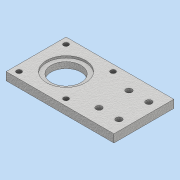
# Autodesk Inventor part: Uchwyt silnika krokowego osi Y - płaski
Saved by Autodesk Inventor 2018 (Build 220112000, 112)
## iProperties
Created: 2019-01-31
Part Number: Uchwyt silnika krokowego osi Y - płaski
Material: Ogólny
Document SubType Name: Modeling
Designer: Dawid
Density: 1 g/cm^3
Appearance: Aluminium odlewane
Author: Dawid
Autodesk Inventor part; units mm, degrees
ref_plane "YZ Plane" through (0, 0, 0) normal (1, 0, 0) x (0, 1, 0)
ref_plane "XZ Plane" through (0, 0, 0) normal (0, 1, 0) x (-1, 0, 0)
ref_plane "XY Plane" through (0, 0, 0) normal (0, 0, 1) x (1, 0, 0)
sketch "Szkic1" plane through (0, 0, 0) normal (0, 0, 1) x (1, 0, 0)
  circle A0 centre (30, 30) radius 15
  circle A1 centre (53.57, 6.43) radius 2.5
  circle A2 centre (6.43, 53.57) radius 2.5
  circle A3 centre (6.43, 6.43) radius 2.5
  circle A4 centre (53.57, 53.57) radius 2.5
  line L0 (0, 60) -> (0, 0)
  line L1 (0, 0) -> (78, 0)
  circle A5 centre (78, 45) radius 3
  circle A6 centre (98, 45) radius 3
  circle A7 centre (98, 15) radius 3
  circle A8 centre (78, 15) radius 3
  line L2 (108, 60) -> (108, 0)
  line L3 (0, 60) -> (108, 60)
  line L4 (108, 0) -> (78, 0)
  point P0 (35, 30)
  dimension "d12" = 6.43
  dimension "d13" = 6.43
  dimension "d14" = 47.14
  dimension "d15" = 47.14
  dimension "d16" = 30
  dimension "d17" = 10
  dimension "d18" = 10
  dimension "d19" = 30
  dimension "d20" = 30
  dimension "d21" = 108
  constraints: 10 end point, 9 centre point, 1 horizontal, 1 parallel
  measures "d12" distance from line of L0 A2.centre
  measures "d13" distance from line of L0 A3.centre
  measures "d14" distance of A2.centre A4.centre
  measures "d15" distance of A1.centre A3.centre
  measures "d16" distance from line of L2 A5.centre
  measures "d17" distance from line of L2 A6.centre
  measures "d18" distance from line of L2 A7.centre
  measures "d19" distance from line of L2 A8.centre
  measures "d20" distance from line of L0 A0.centre
  measures "d21" distance of L0.start L2.start
extrude "Wyciągnięcie proste1" add sketch "Szkic1" along normal blind 8
thread "Gwint1" size "M5x0.8" class "6H" standard "ANSI Metric M Profile" full length
thread "Gwint2" size "M5x0.8" class "6H" standard "ANSI Metric M Profile" full length
thread "Gwint3" size "M5x0.8" class "6H" standard "ANSI Metric M Profile" full length
thread "Gwint4" size "M5x0.8" class "6H" standard "ANSI Metric M Profile" full length
sketch "Szkic2" plane through (0, 0, 8) normal (0, 0, 1) x (1, 0, 0)
  circle A0 centre (30, 30) radius 19.5
  circle A1 centre (53.57, 53.57) radius 2.5
  circle A2 centre (6.43, 6.43) radius 2.5
  circle A3 centre (6.43, 53.57) radius 2.5
  circle A4 centre (53.57, 6.43) radius 2.5
  line L0 (70, 60) -> (70, 0)
  line L1 (0, 60) -> (70, 60)
  line L2 (0, 0) -> (0, 60)
  line L3 (70, 0) -> (0, 0)
  circle A5 centre (30, 30) radius 15
  circle A6 centre (30, 30) radius 19.5
  circle A7 centre (30, 30) radius 15 projected
  circle A8 centre (78, 15) radius 3 projected
  circle A9 centre (98, 15) radius 3 projected
  circle A10 centre (98, 45) radius 3 projected
  circle A11 centre (78, 45) radius 3 projected
  circle A12 centre (53.57, 53.57) radius 2.5 projected
  circle A13 centre (6.43, 6.43) radius 2.5 projected
  circle A14 centre (6.43, 53.57) radius 2.5 projected
  circle A15 centre (53.57, 6.43) radius 2.5 projected
  line L4 (0, 60) -> (0, 0) projected
  line L5 (0, 0) -> (108, 0) projected
  line L6 (108, 0) -> (108, 60) projected
  line L7 (108, 60) -> (0, 60) projected
  point P0 (35, 30)
  constraints: 8 end point, 7 centre point
extrude "Wyciągnięcie proste2" cut sketch "Szkic2" against normal blind 2 contours A0
